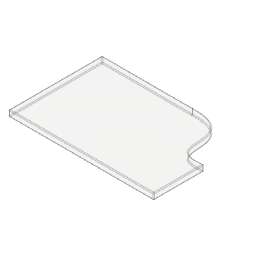
_ESP Lid With Hook.bd890dbd-94a6-4cf6-a228-404acde44ffc (Autodesk Fusion 360 design; units mm, degrees)
Autodesk Fusion 360 part; units mm, degrees
sketch "sketch 648" plane through (0, 0, 27) normal (0, 0, 1) x (-1, 0, 0)
  line L0 (-147.2888, 46.26) -> (-89.44, 46.26)
  line L1 (-89.44, 46.26) -> (-89.44, 106.14)
  line L2 (-89.44, 106.14) -> (-182.34, 106.14)
  line L3 (-182.34, 106.14) -> (-182.34, 74.0043)
  spline S0 degree 3 poles (-147.2888, 46.26) (-150.6096, 46.1574) (-153.7082, 46.3347) (-159.1015, 47.5278) (-160.782, 48.3635) (-163.103, 49.7634) (-164.2633, 50.7604) (-165.9986, 52.9987) (-166.8009, 54.401) (-168.2255, 59.3639) (-168.2987, 62.4706) (-168.66, 66.8403) (-168.8443, 68.4419) (-169.5239, 70.5051) (-169.8364, 71.2154) (-170.7326, 72.3831) (-171.2152, 72.811) (-172.4466, 73.5137) (-173.3583, 73.9081) (-177.2522, 74.516) (-179.3167, 74.2869) (-182.34, 74.0043) knots -14.954017 -14.954017 -14.954017 -14.954017 -13.094513 -13.094513 -11.321554 -11.321554 -9.035694 -9.035694 -7.073539 -7.073539 -4.267631 -4.267631 -2.775762 -2.775762 -2.059383 -2.059383 -1.476586 -1.476586 -0.910958 -0.910958 0 0 0 0
extrude "Extrude1" add sketch "sketch 648" along normal blind 4
fillet "Fillet1" radius 0.5 1 edges at (135.89, -106.14, 31) 6 faces at (120.4067, -106.14, 28.3333) (108.7229, -66.22, 31) (182.34, -95.4281, 28.3333) (168.3486, -62.799, 28.3333) (128.0059, -46.26, 28.3333) (89.44, -66.22, 28.3333)
extrude "Extrude2" [rolled back] along distance 12 taper angle 0
extrude "Extrude3" [rolled back] along distance -7 taper angle 0
extrude "Extrude4" [rolled back] along distance -7 taper angle 0
extrude "Extrude5" [rolled back] along distance -7 taper angle 0
extrude "Extrude6" [rolled back] along distance -7 taper angle 0
